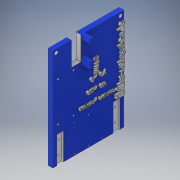
# Autodesk Inventor part: MainBody
Saved by Autodesk Inventor 2018 (Build 220112000, 112)
## iProperties
Created: 2018-10-10
Part Number: MainBody
Material: Generic
Document SubType Name: Modeling
Designer: Viraj Shah
Density: 1 g/cm^3
Appearance: Default
Author: Viraj Shah
Autodesk Inventor part; units mm, degrees
ref_plane "YZ Plane" through (0, 0, 0) normal (1, 0, 0) x (0, 1, 0)
ref_plane "XZ Plane" through (0, 0, 0) normal (0, 1, 0) x (-1, 0, 0)
ref_plane "XY Plane" through (0, 0, 0) normal (0, 0, 1) x (1, 0, 0)
sketch "Sketch1" plane through (0, 0, 0) normal (1, 0, 0) x (0, 1, 0)
  line L0 (50, -400.7355) -> (-50, -400.7355)
  line L1 (-50, -400.7355) -> (-50, -430.7355)
  line L2 (-50, -430.7355) -> (50, -430.7355)
  line L3 (50, -430.7355) -> (50, -400.7355)
  line L4 (-52.5, -305.7355) -> (52.5, -305.7355)
  line L5 (52.5, -305.7355) -> (52.5, -455.7355)
  line L6 (52.5, -455.7355) -> (-52.5, -455.7355)
  line L7 (-52.5, -455.7355) -> (-52.5, -305.7355)
  dimension "d4" = 100
  dimension "d5" = 30
  dimension "d7" = 105
  dimension "d8" = 150
  dimension "d9" = 2.5
  dimension "d10" = 55
  constraints: 16 end point, 4 parallel, 2 perpendicular, 1 horizontal
  measures "d4" distance of L3.start L2.start
  measures "d5" distance of L2.start L0.end
  measures "d7" distance of L5.end L6.end
  measures "d8" distance of L4.end L5.end
  measures "d9" distance between parallel lines of L7 L1
  measures "d10" distance between parallel lines of L6 L0
extrude "Extrusion1" add sketch "Sketch1" along normal blind 7 contours L3 L2 L1 L0 | L4 L5 L6 L7
sketch "Sketch3" plane through (0, -52.5, -455.7355) normal (0, 0, -1) x (-1, 0, 0)
  line L0 (0, 0) -> (-7, 0) projected
  line L1 (-7, 0) -> (-7, 105) projected
  line L2 (-7, 6) -> (-4.5, 6)
  line L3 (-4.5, 6) -> (-4.5, 16)
  line L4 (-4.5, 16) -> (-7, 16)
  line L5 (-7, 6) -> (-7, 16)
  line L6 (0, 52.5) -> (-22.4318, 52.5)
  line L7 (-7, 99) -> (-4.5, 99)
  line L8 (-4.5, 99) -> (-4.5, 89)
  line L9 (-4.5, 89) -> (-7, 89)
  line L10 (-7, 99) -> (-7, 89)
  dimension "d19" = 6
  dimension "d20" = 2.5
  dimension "d21" = 10
  constraints: 18 end point, 4 symmetric about line, 2 horizontal, 2 perpendicular, 2 point on line
  measures "d19" distance of L0.end L2.start
  measures "d20" distance of L2.start L2.end
  measures "d21" distance of L2.end L3.end
extrude "Extrusion3" cut sketch "Sketch3" against normal blind 40
sketch "Sketch4" plane through (7, 0, 0) normal (1, 0, 0) x (0, 0, -1)
  line L0 (305.7355, -52.5) -> (455.7355, -52.5) projected
  line L1 (305.7355, 52.5) -> (305.7355, -52.5) projected
  line L2 (455.7355, 52.5) -> (305.7355, 52.5) projected
  circle A0 centre (310.7355, 47.5) radius 2.5
  circle A1 centre (310.7355, -47.5) radius 2.5
  point P0 (0, 0)
  dimension "d24" = 5
  dimension "d25" = 5
  dimension "d26" = 5
  dimension "d27" = 5
  dimension "d28" = 5
  dimension "d29" = 5
  constraints: 2 centre point, 2 coincident
  measures "d24" distance from line of L0 point (310.736, -47.5)
  measures "d25" distance from line of L1 point (310.736, -47.5)
  measures "d26" distance from line of L2 point (310.736, 47.5)
  measures "d27" distance from line of L1 point (310.736, 47.5)
  measures "d28" diameter of A0
  measures "d29" diameter of A1
extrude "Extrusion4" cut sketch "Sketch4" against normal blind 40
sketch "Sketch5" plane through (7, 0, 0) normal (1, 0, 0) x (0, 0, -1)
  line L0 (305.7355, -52.5) -> (455.7355, -52.5) projected
  line L1 (305.7355, 52.5) -> (305.7355, -52.5) projected
  circle A0 centre (345.7355, -44.85) radius 1.375
  circle A1 centre (345.7355, -21.85) radius 1.375
  circle A2 centre (403.7355, -21.85) radius 1.375
  circle A3 centre (403.7355, -44.85) radius 1.375
  point P0 (0, 0)
  dimension "d32" = 23
  dimension "d34" = 58
  dimension "d35" = 7.65
  dimension "d36" = 7.65
  dimension "d37" = 0
  dimension "d38" = 58
  dimension "d39" = 40
  dimension "d40" = 2.75
  dimension "d41" = 2.75
  dimension "d42" = 2.75
  dimension "d43" = 2.75
  dimension "d111" = 23
  constraints: 4 centre point, 4 coincident
  measures "d32" distance of point (345.736, -21.85) point (345.736, -44.85)
  measures "d34" distance of point (345.736, -44.85) point (403.736, -44.85)
  measures "d35" distance from line of L0 point (345.736, -44.85)
  measures "d36" distance from line of L0 point (403.736, -44.85)
  measures "d37" horizontal distance of point (403.736, -21.85) point (403.736, -44.85)
  measures "d38" distance of point (403.736, -21.85) point (345.736, -21.85)
  measures "d39" distance from line of L1 point (345.736, -21.85)
  measures "d40" diameter of A0
  measures "d41" diameter of A1
  measures "d42" diameter of A2
  measures "d43" diameter of A3
  measures "d111" distance of point (403.736, -21.85) point (403.736, -44.85)
extrude "Extrusion5" cut sketch "Sketch5" against normal blind 40
sketch "Sketch6" plane through (7, 0, 0) normal (1, 0, 0) x (0, 0, -1)
  line L0 (0, 0) -> (765.3396, 0)
  line L1 (305.7355, -25) -> (340.7355, -25)
  line L2 (305.7355, -11) -> (340.7355, -11)
  line L3 (340.7355, -11) -> (340.7355, -25)
  line L4 (305.7355, -25) -> (305.7355, -11)
  constraints: 10 end point, 1 horizontal
extrude "Extrusion6" cut sketch "Sketch6" against normal blind 40
sketch "Sketch7" plane through (7, 0, 0) normal (1, 0, 0) x (0, 0, -1)
  line L0 (305.7355, 52.5) -> (305.7355, -11) projected
  line L1 (305.7355, -10) -> (311.7355, -10)
  line L2 (311.7355, -10) -> (311.7355, -5)
  line L3 (311.7355, -5) -> (305.7355, -5)
  line L4 (305.7355, -5) -> (305.7355, -10)
  line L5 (305.7355, -11) -> (340.7355, -11) projected
  line L6 (335.2355, -10) -> (344.2355, -10)
  line L7 (344.2355, -10) -> (344.2355, -5)
  line L8 (344.2355, -5) -> (335.2355, -5)
  line L9 (335.2355, -5) -> (335.2355, -10)
  point P0 (0, 0)
  dimension "d54" = 6
  dimension "d55" = 5
  dimension "d56" = 1
  dimension "d57" = 9
  dimension "d58" = 5
  dimension "d59" = 23.5
  dimension "d73" = 0
  constraints: 16 end point, 4 parallel, 2 horizontal, 2 perpendicular, 1 point on line
  measures "d54" distance of L3.end L2.end
  measures "d55" distance of L2.end L1.end
  measures "d56" distance between parallel lines of L5 L1
  measures "d57" distance of L8.end L7.end
  measures "d58" distance of L7.end L6.end
  measures "d59" distance between parallel lines of L9 L2
  measures "d73" distance between parallel lines of L6 L1
extrude "Extrusion7" add sketch "Sketch7" along normal blind 12
sketch "Sketch8" plane through (7, -10, -344.2355) normal (0, -1, 0) x (1, 0, 0)
  line L0 (12, 38.5) -> (12, 32.5) projected
  line L1 (12, 9) -> (12, 0) projected
  line L2 (0, 9) -> (12, 9) projected
  point P0 (-7, 344.2355)
  point P1 (6, 6.5)
  point P2 (6, 35.5)
  dimension "d62" = 6
  dimension "d63" = 6
  dimension "d64" = 2.5
  dimension "d65" = 29
  measures "d62" distance from line of L0 point (6, 35.5)
  measures "d63" distance from line of L1 point (6, 6.5)
  measures "d64" distance from line of L2 point (6, 6.5)
  measures "d65" distance of point (6, 35.5) point (6, 6.5)
hole "Hole1" [suppressed]
sketch "Sketch10" plane through (4.5, -46.5, -455.7355) normal (1, 0, 0) x (0, 0, -1)
  line L0 (0, 0) -> (-40, 0) projected
  line L1 (0, 99) -> (0, -6) projected
  circle A0 centre (-30, 5) radius 1
  circle A1 centre (-10, 5) radius 1
  line L2 (0, 10) -> (0, 83) projected
  line L3 (0, 46.5) -> (-66.3883, 46.5)
  circle A2 centre (-30, 88) radius 1
  circle A3 centre (-10, 88) radius 1
  point P0 (-455.7355, 46.5)
  dimension "d77" = 2
  dimension "d78" = 2
  constraints: 4 centre point, 4 coincident, 4 symmetric about line, 2 end point, 1 horizontal, 1 midpoint, 2 other
  measures "d77" diameter of A0
  measures "d78" diameter of A1
extrude "Extrusion8" cut sketch "Sketch10" against normal blind 10
sketch "Sketch11" plane through (7, 0, 0) normal (1, 0, 0) x (0, 0, -1)
  circle A0 centre (369.0216, 10.3693) radius 3.1
  circle A1 centre (384.0216, 10.3693) radius 3.1
  circle A2 centre (399.0216, 10.3693) radius 3.1
  point P0 (0, 0)
  dimension "d83" = 15
  dimension "d84" = 15
  dimension "d85" = 6.2
  dimension "d86" = 6.2
  dimension "d87" = 6.2
  constraints: 3 centre point, 3 coincident
  measures "d83" distance of point (384.022, 10.369) point (369.022, 10.369)
  measures "d84" distance of point (384.022, 10.369) point (399.022, 10.369)
  measures "d85" diameter of A0
  measures "d86" diameter of A1
  measures "d87" diameter of A2
extrude "Extrusion9" cut sketch "Sketch11" against normal blind 10
sketch "Sketch12" plane through (7, 0, 0) normal (1, 0, 0) x (0, 0, -1)
  line L0 (305.7355, 52.5) -> (455.7355, 52.5) projected
  line L1 (389.0354, 35.8376) -> (378.0354, 35.8376)
  line L2 (378.0354, 38.8376) -> (382.0354, 38.8376)
  line L3 (382.0354, 38.8376) -> (382.0354, 47.8376)
  line L4 (382.0354, 47.8376) -> (378.0354, 47.8376)
  line L5 (389.0354, 38.8376) -> (385.0354, 38.8376)
  line L6 (385.0354, 38.8376) -> (385.0354, 47.8376)
  line L7 (385.0354, 47.8376) -> (389.0354, 47.8376)
  line L8 (373.0515, 35.8462) -> (373.0946, 50.8376)
  line L9 (370.0702, 42.3462) -> (364.3334, 35.8376)
  line L10 (364.3334, 35.8376) -> (362.9588, 37.6685)
  line L11 (370.0759, 44.3462) -> (364.3766, 50.8877)
  line L12 (364.3766, 50.8877) -> (362.9915, 49.0648)
  line L13 (370.0515, 35.8462) -> (370.0702, 42.3462)
  line L14 (370.0759, 44.3462) -> (370.0946, 50.8462)
  line L15 (362.3922, 38.3188) -> (366.8317, 43.3555)
  line L16 (366.8317, 43.3555) -> (362.4632, 48.3694)
  line L17 (369.2394, 50.8376) -> (369.2395, 50.8487)
  line L18 (362.9915, 49.0648) -> (362.4632, 48.3694)
  line L19 (362.9588, 37.6685) -> (362.3922, 38.3188)
  line L20 (347.6585, 38.8376) -> (351.6582, 38.8376)
  line L21 (351.6582, 38.8376) -> (351.6582, 47.8376)
  line L22 (351.6582, 47.8376) -> (347.6585, 47.8376)
  line L23 (358.6585, 38.8376) -> (354.6582, 38.8376)
  line L24 (354.6582, 38.8376) -> (354.6582, 47.8376)
  line L25 (354.6582, 47.8376) -> (358.6585, 47.8376)
  line L26 (391.0354, 35.8376) -> (391.0354, 35.8462)
  line L27 (378.0354, 50.8376) -> (389.0354, 50.8376)
  line L28 (370.0945, 50.8376) -> (373.0946, 50.8376)
  line L29 (364.3386, 50.8376) -> (364.4202, 50.8376)
  line L30 (389.0354, 35.8376) -> (378.0354, 35.8376)
  line L31 (373.0515, 35.8462) -> (370.0515, 35.8462)
  line L32 (358.6585, 35.8376) -> (347.6585, 35.8376)
  line L33 (358.6585, 50.8376) -> (347.6585, 50.8376)
  line L34 (389.0354, 35.8376) -> (389.0354, 38.8376)
  line L35 (389.0354, 47.8376) -> (389.0354, 50.8376)
  line L36 (378.0354, 35.8376) -> (378.0354, 38.8376)
  line L37 (378.0354, 47.8376) -> (378.0354, 50.8376)
  line L38 (376.0354, 35.8376) -> (376.0354, 35.8462)
  line L39 (358.6585, 35.8376) -> (358.6585, 38.8376)
  line L40 (358.6585, 47.8376) -> (358.6585, 50.8376)
  line L41 (347.6585, 35.8376) -> (347.6585, 38.8376)
  line L42 (347.6585, 47.8376) -> (347.6585, 50.8376)
  point P0 (0, 0)
  constraints: 84 end point, 14 parallel, 7 perpendicular, 5 point on line, 3 horizontal
extrude "Extrusion10" [suppressed]
sketch "Sketch14" plane through (7, 0, 0) normal (1, 0, 0) x (0, 0, -1)
  circle A0 centre (399.0216, 10.3693) radius 3.1 projected
  line L0 (383.5696, 16.8077) -> (384.0734, 16.8077) construction
  line L1 (383.5696, 14.7372) -> (384.0734, 14.7372)
  line L2 (384.0734, 18.8783) -> (383.5696, 18.8783)
  arc A1 (383.5696, 18.8783) -> (383.5696, 14.7372) centre (383.5696, 16.8077) ccw
  arc A2 (384.0734, 14.7372) -> (384.0734, 18.8783) centre (384.0734, 16.8077) ccw
  line L3 (384.0734, 16.1243) -> (383.5696, 16.1243)
  arc A3 (383.5696, 17.4911) -> (383.5696, 16.1243) centre (383.5696, 16.8077) ccw
  line L4 (383.5696, 17.4911) -> (384.0734, 17.4911)
  arc A4 (384.0734, 16.1243) -> (384.0734, 17.4911) centre (384.0734, 16.8077) ccw
  line L5 (386.247, 19.4647) -> (381.907, 19.4647)
  line L6 (386.247, 20.5147) -> (383.3413, 20.5147)
  line L7 (381.907, 20.7247) -> (384.4441, 22.1895)
  line L8 (386.1241, 22.1895) -> (384.5223, 21.2647)
  line L9 (386.1241, 23.2395) -> (381.802, 23.2395)
  line L10 (384.4441, 22.1895) -> (381.802, 22.1895)
  line L11 (384.5223, 21.2647) -> (383.3413, 20.5147)
  line L12 (386.247, 19.4647) -> (386.247, 20.5147)
  line L13 (386.1241, 22.1895) -> (386.1241, 23.2395)
  line L14 (381.907, 19.4647) -> (381.907, 20.7247)
  line L15 (381.802, 22.1895) -> (381.802, 23.2395)
  circle A5 centre (384.0216, 10.3693) radius 3.1 projected
  line L16 (386.1316, 3.7704) -> (381.4806, 3.7704)
  line L17 (381.4806, 6.4304) -> (382.3206, 6.4304)
  line L18 (382.3206, 6.4304) -> (382.3206, 4.6104)
  line L19 (382.3206, 4.6104) -> (383.1606, 4.6104)
  line L20 (383.1606, 4.6104) -> (383.1606, 5.8704)
  line L21 (384.0006, 5.8704) -> (384.0006, 4.6104)
  line L22 (384.0006, 4.6104) -> (386.1316, 4.6104)
  line L23 (386.1316, 3.7704) -> (386.1316, 4.6104)
  line L24 (381.4806, 6.4304) -> (381.4806, 3.7704)
  line L25 (383.1606, 5.8704) -> (384.0006, 5.8704)
  line L26 (381.4806, 3.4273) -> (382.3206, 3.4273)
  line L27 (382.3206, 1.6073) -> (383.1606, 1.6073)
  line L28 (384.0006, 2.8673) -> (384.0006, 1.6073)
  line L29 (383.1606, 1.6073) -> (383.1606, 2.8673)
  line L30 (382.3206, 3.4273) -> (382.3206, 1.6073)
  line L31 (384.0006, 1.6073) -> (386.1316, 1.6073)
  line L32 (386.1316, 0.7673) -> (381.4806, 0.7673)
  line L33 (386.1316, 0.7673) -> (386.1316, 1.6073)
  line L34 (381.4806, 3.4273) -> (381.4806, 0.7673)
  line L35 (383.1606, 2.8673) -> (384.0006, 2.8673)
  line L36 (397.327, -12.2248) -> (397.975, -12.2248)
  line L37 (397.975, -13.6288) -> (398.623, -13.6288)
  line L38 (399.271, -12.6568) -> (399.271, -13.6288)
  line L39 (398.623, -13.6288) -> (398.623, -12.6568)
  line L40 (397.975, -12.2248) -> (397.975, -13.6288)
  line L41 (399.271, -13.6288) -> (400.9149, -13.6288)
  line L42 (400.9149, -14.2768) -> (397.327, -14.2768)
  line L43 (400.9149, -14.2768) -> (400.9149, -13.6288)
  line L44 (397.327, -12.2248) -> (397.327, -14.2768)
  line L45 (398.623, -12.6568) -> (399.271, -12.6568)
  line L46 (400.9651, -8.0846) -> (397.2712, -8.0846)
  arc A6 (399.1232, -6.8327) -> (397.2712, -6.8342) centre (398.1975, -7.1989) ccw
  line L47 (399.1232, -6.8327) -> (401.0087, -6.0517)
  line L48 (399.374, -7.3782) -> (401.0087, -6.7011)
  line L49 (400.9651, -7.4846) -> (399.374, -7.4846)
  line L50 (399.374, -7.3782) -> (399.374, -7.4846)
  line L51 (397.297, -5.8571) -> (400.9651, -5.8571)
  line L52 (397.297, -5.2571) -> (400.4972, -5.2571)
  line L53 (400.9651, -4.8344) -> (399.5174, -3.9985)
  line L54 (400.9651, -4.8344) -> (402.6367, -4.8344) construction
  line L55 (400.4972, -5.2571) -> (398.2454, -3.957)
  line L56 (397.297, -2.1024) -> (400.9651, -2.1024)
  line L57 (397.297, -2.6569) -> (400.4972, -2.6569)
  line L58 (400.9651, -3.1627) -> (399.5174, -3.9985)
  line L59 (400.4972, -2.6569) -> (398.2454, -3.957)
  line L60 (400.9651, -1.8466) -> (397.327, -0.3767)
  line L61 (400.9651, -1.2642) -> (399.6523, -0.7338)
  line L62 (400.9651, 0.8232) -> (397.327, -0.3767)
  line L63 (400.9651, 0.2546) -> (399.6523, -0.1784)
  line L64 (399.6523, -0.7338) -> (399.6523, -0.1784)
  line L65 (400.9371, 1.2698) -> (397.2991, 1.2698)
  arc A7 (399.1511, 2.5217) -> (397.2991, 2.5201) centre (398.2254, 2.1554) ccw
  line L66 (399.1511, 2.5217) -> (401.0366, 3.3027)
  line L67 (399.4019, 1.9761) -> (401.0366, 2.6532)
  line L68 (400.9371, 1.8698) -> (399.4019, 1.8698)
  line L69 (399.4019, 1.9761) -> (399.4019, 1.8698)
  line L70 (400.9651, 3.7854) -> (397.327, 3.7854)
  arc A8 (400.9651, 3.7854) -> (397.327, 3.7854) centre (399.146, 4.0442) ccw
  line L71 (400.9651, -8.0846) -> (400.9651, -7.4846)
  line L72 (401.0087, -6.7011) -> (401.0087, -6.0517)
  line L73 (400.9651, -5.8571) -> (400.9651, -4.8344)
  line L74 (400.9651, -3.1627) -> (400.9651, -2.1024)
  line L75 (400.9651, -1.8466) -> (400.9651, -1.2642)
  line L76 (400.9651, 0.2546) -> (400.9651, 0.8232)
  line L77 (400.9371, 1.2698) -> (400.9371, 1.8698)
  line L78 (401.0366, 2.6532) -> (401.0366, 3.3027)
  line L79 (397.2712, -8.0846) -> (397.2712, -6.8342)
  line L80 (397.297, -5.8571) -> (397.297, -5.2571)
  line L81 (397.297, -2.6569) -> (397.297, -2.1024)
  line L82 (397.2991, 1.2698) -> (397.2991, 2.5201)
  line L83 (397.3471, 24.6024) -> (401.0152, 24.6024)
  line L84 (397.3471, 25.2024) -> (400.5474, 25.2024)
  line L85 (401.0152, 25.6252) -> (399.5675, 26.461)
  line L86 (401.0152, 25.6252) -> (402.6869, 25.6252) construction
  line L87 (400.5474, 25.2024) -> (398.2955, 26.5026)
  line L88 (397.3471, 28.3572) -> (401.0152, 28.3572)
  line L89 (397.3471, 27.8027) -> (400.5474, 27.8027)
  line L90 (400.5474, 27.8027) -> (398.2955, 26.5026)
  line L91 (401.0152, 27.2968) -> (399.5675, 26.461)
  line L92 (401.0152, 28.613) -> (397.3771, 30.0828)
  line L93 (401.0152, 29.1954) -> (399.7025, 29.7257)
  line L94 (401.0152, 31.2828) -> (397.3771, 30.0828)
  line L95 (401.0152, 30.7142) -> (399.7025, 30.2812)
  line L96 (399.7025, 29.7257) -> (399.7025, 30.2812)
  arc A9 (399.2012, 32.7656) -> (397.3492, 32.764) centre (398.2755, 32.3993) ccw
  line L97 (399.4521, 32.22) -> (399.4521, 32.1137)
  line L98 (400.9873, 31.5137) -> (397.3492, 31.5137)
  line L99 (399.2012, 32.7656) -> (401.0867, 33.5466)
  line L100 (399.4521, 32.22) -> (401.0867, 32.8971)
  line L101 (400.9873, 32.1137) -> (399.4521, 32.1137)
  line L102 (401.0152, 34.2449) -> (397.3771, 34.2449)
  arc A10 (401.0152, 34.2449) -> (397.3771, 34.2449) centre (399.1962, 34.5038) ccw
  line L103 (401.0152, 24.6024) -> (401.0152, 25.6252)
  line L104 (401.0152, 27.2968) -> (401.0152, 28.3572)
  line L105 (401.0152, 28.613) -> (401.0152, 29.1954)
  line L106 (401.0152, 30.7142) -> (401.0152, 31.2828)
  line L107 (400.9873, 31.5137) -> (400.9873, 32.1137)
  line L108 (401.0867, 32.8971) -> (401.0867, 33.5466)
  line L109 (397.3471, 24.6024) -> (397.3471, 25.2024)
  line L110 (397.3471, 27.8027) -> (397.3471, 28.3572)
  line L111 (397.3492, 31.5137) -> (397.3492, 32.764)
  arc A11 (399.1962, 16.0661) -> (397.3771, 16.0699) centre (398.286, 15.7439) ccw
  line L112 (397.3771, 14.8176) -> (397.3771, 16.0699)
  line L113 (399.1962, 14.8176) -> (397.3771, 14.8176)
  line L114 (399.1962, 14.8176) -> (401.0152, 14.8176)
  arc A12 (401.0152, 16.0699) -> (399.1962, 16.0661) centre (400.1064, 15.7439) ccw
  line L115 (401.0152, 16.7094) -> (401.0152, 17.2918)
  line L116 (401.0152, 16.7094) -> (397.3771, 18.1793)
  line L117 (401.0152, 17.2918) -> (399.7025, 17.8222)
  line L118 (401.0152, 19.3792) -> (397.3771, 18.1793)
  line L119 (401.0152, 18.8106) -> (399.7025, 18.3776)
  line L120 (399.7025, 17.8222) -> (399.7025, 18.3776)
  line L121 (401.0152, 18.8106) -> (401.0152, 19.3792)
  arc A13 (397.4543, 21.4637) -> (400.9493, 21.4059) centre (399.1937, 20.9472) ccw
  arc A14 (398.3792, 20.9472) -> (400.0082, 20.9472) centre (399.1937, 20.9472) ccw
  line L122 (398.3792, 20.9472) -> (398.3792, 21.4637)
  line L123 (400.0082, 20.9472) -> (400.0082, 21.4059)
  line L124 (397.4543, 21.4637) -> (398.3792, 21.4637)
  line L125 (400.0082, 21.4059) -> (400.9493, 21.4059)
  line L126 (397.3771, 21.9899) -> (401.0152, 21.9899)
  line L127 (398.6702, 22.5899) -> (397.3771, 23.883)
  line L128 (397.8014, 24.3073) -> (399.3091, 22.7996)
  line L129 (399.948, 22.5899) -> (401.0152, 23.6571)
  line L130 (400.5909, 24.0814) -> (399.3091, 22.7996)
  line L131 (397.3771, 22.5899) -> (398.6702, 22.5899)
  line L132 (399.948, 22.5899) -> (401.0152, 22.5899)
  line L133 (401.0152, 23.6571) -> (400.5909, 24.0814)
  line L134 (397.3771, 23.883) -> (397.8014, 24.3073)
  line L135 (401.0152, 22.5899) -> (401.0152, 21.9899)
  line L136 (397.3771, 22.5899) -> (397.3771, 21.9899)
  circle A15 centre (369.0216, 10.3693) radius 3.1 projected
  line L137 (365.9216, 23.083) -> (365.9216, 23.9821)
  line L138 (368.4931, 16.6306) -> (369.1625, 16.6306) construction
  line L139 (368.5036, 14.5059) -> (369.173, 14.5092)
  line L140 (369.152, 18.7587) -> (368.4826, 18.7554)
  line L141 (368.4897, 17.3185) -> (369.03, 17.3212)
  line L142 (369.0055, 15.9453) -> (368.4965, 15.9428)
  arc A16 (368.4897, 17.3185) -> (368.4965, 15.9428) centre (368.4931, 16.6306) ccw
  arc A17 (369.0055, 15.9453) -> (369.03, 17.3212) centre (369.1625, 16.6306) ccw
  arc A18 (368.4826, 18.7554) -> (368.5036, 14.5059) centre (368.4931, 16.6306) ccw
  arc A19 (369.173, 14.5092) -> (371.2812, 16.5222) centre (369.1625, 16.6306) ccw
  arc A20 (370.9611, 17.7681) -> (369.152, 18.7587) centre (369.1625, 16.6306) ccw
  line L143 (371.2812, 16.5222) -> (372.4335, 18.518)
  line L144 (371.2812, 16.5222) -> (373.5859, 16.5222) construction
  line L145 (370.9611, 17.7681) -> (371.8272, 19.2681)
  line L146 (370.9611, 17.7681) -> (372.6932, 17.7681) construction
  line L147 (372.4335, 18.518) -> (371.8272, 19.2681)
  line L148 (372.1216, 19.9028) -> (365.9216, 23.083)
  line L149 (372.1216, 23.9686) -> (369.7794, 22.0033)
  line L150 (372.1216, 24.3698) -> (374.6501, 24.3698) construction
  line L151 (372.1216, 25.0129) -> (369.007, 22.3995)
  line L152 (372.1216, 19.9028) -> (372.1216, 20.8019)
  line L153 (372.1216, 23.9686) -> (372.1216, 25.0129)
  line L154 (372.1216, 20.8019) -> (369.7794, 22.0033)
  line L155 (369.007, 22.3995) -> (365.9216, 23.9821)
  arc A21 (368.8932, 3.7279) -> (368.9, 2.3522) centre (368.8966, 3.0401) ccw
  line L156 (368.9071, 0.9153) -> (369.5765, 0.9186)
  line L157 (369.409, 2.3547) -> (368.9, 2.3522)
  line L158 (368.8966, 3.0401) -> (369.566, 3.0401) construction
  line L159 (368.8932, 3.7279) -> (369.4335, 3.7306)
  arc A22 (369.409, 2.3547) -> (369.4335, 3.7306) centre (369.566, 3.0401) ccw
  arc A23 (368.8861, 5.1648) -> (368.9071, 0.9153) centre (368.8966, 3.0401) ccw
  line L160 (369.5555, 5.1681) -> (368.8861, 5.1648)
  line L161 (372.5251, 4.42) -> (372.5251, 5.4504)
  arc A24 (369.5765, 0.9186) -> (371.6847, 2.9316) centre (369.566, 3.0401) ccw
  arc A25 (371.3646, 4.1775) -> (369.5555, 5.1681) centre (369.566, 3.0401) ccw
  line L162 (371.6847, 2.9316) -> (372.837, 4.9274)
  line L163 (371.6847, 2.9316) -> (373.9893, 2.9316) construction
  line L164 (371.3646, 4.1775) -> (372.2306, 5.6775)
  line L165 (371.3646, 4.1775) -> (373.0967, 4.1775) construction
  line L166 (372.837, 4.9274) -> (372.2306, 5.6775)
  line L167 (360.9007, 12.9625) -> (358.6077, 7.2872)
  line L168 (359.9921, 12.9625) -> (359.1647, 10.9147)
  line L169 (356.7358, 12.9625) -> (358.6077, 7.2872)
  line L170 (357.6228, 12.9625) -> (358.2982, 10.9147)
  line L171 (359.1647, 10.9147) -> (358.2982, 10.9147)
  line L172 (360.9007, 12.9625) -> (359.9921, 12.9625)
  line L173 (357.6228, 12.9625) -> (356.7358, 12.9625)
  line L174 (364.5611, 7.2699) -> (363.5675, 12.9956)
  line L175 (363.2589, 7.2699) -> (362.5002, 11.6419)
  line L176 (362.5002, 13.2978) -> (367.8961, 13.2978) construction
  line L177 (360.4301, 7.2764) -> (361.3567, 12.9956)
  line L178 (361.7296, 7.2764) -> (362.5002, 11.6419)
  line L179 (356.3334, 7.2699) -> (356.3334, 12.9956)
  line L180 (352.6489, 12.9956) -> (352.6489, 11.9386)
  line L181 (352.6489, 11.9386) -> (355.12, 11.9386)
  line L182 (355.12, 11.9386) -> (355.12, 7.2699)
  line L183 (355.12, 11.9386) -> (361.2012, 11.9386) construction
  line L184 (351.4679, 7.2699) -> (351.4679, 11.6838)
  line L185 (348.4679, 7.2699) -> (348.4679, 11.6838)
  arc A26 (351.4679, 11.6838) -> (348.4679, 11.6838) centre (349.9679, 11.0315) ccw
  line L186 (347.4679, 7.2699) -> (347.4679, 11.8664)
  arc A27 (352.4679, 11.8664) -> (347.4679, 11.8664) centre (349.9679, 11.0315) ccw
  line L187 (352.4679, 11.8664) -> (352.4679, 7.2699)
  line L188 (343.5709, 7.2699) -> (343.5709, 8.3067)
  line L189 (344.2621, 9.3435) -> (344.2621, 9.9435)
  line L190 (345.8173, 8.3067) -> (345.8173, 9.3435)
  line L191 (345.8173, 9.3435) -> (344.2621, 9.3435)
  line L192 (343.5709, 8.3067) -> (345.8173, 8.3067)
  line L193 (343.5709, 7.2699) -> (346.8539, 7.2699)
  line L194 (346.8539, 10.2699) -> (346.8539, 7.2699)
  line L195 (343.5709, 13.0199) -> (343.5709, 11.9831)
  line L196 (344.2621, 10.5435) -> (344.2621, 9.9435)
  line L197 (345.8173, 11.9831) -> (345.8173, 10.5435)
  line L198 (345.8173, 10.5435) -> (344.2621, 10.5435)
  line L199 (343.5709, 11.9831) -> (345.8173, 11.9831)
  line L200 (343.5709, 13.0199) -> (346.8539, 13.0199)
  line L201 (346.8539, 10.2699) -> (346.8539, 13.0199)
  line L202 (356.3334, 7.2699) -> (355.12, 7.2699)
  line L203 (356.3334, 12.9956) -> (352.6489, 12.9956)
  line L204 (352.4679, 7.2699) -> (351.4679, 7.2699)
  line L205 (348.4679, 7.2699) -> (347.4679, 7.2699)
  line L206 (383.5696, -2.0145) -> (384.0734, -2.0145) construction
  line L207 (383.5696, -4.0851) -> (384.0734, -4.0851)
  line L208 (384.0734, 0.0561) -> (383.5696, 0.0561)
  line L209 (383.5696, -1.3311) -> (384.0734, -1.3311)
  line L210 (384.0734, -2.6979) -> (383.5696, -2.6979)
  arc A28 (383.5696, -1.3311) -> (383.5696, -2.6979) centre (383.5696, -2.0145) ccw
  arc A29 (384.0734, -2.6979) -> (384.0734, -1.3311) centre (384.0734, -2.0145) ccw
  arc A30 (384.0734, -4.0851) -> (384.0734, 0.0561) centre (384.0734, -2.0145) ccw
  arc A31 (383.5696, 0.0561) -> (383.5696, -4.0851) centre (383.5696, -2.0145) ccw
  line L211 (398.8521, -10.4106) -> (399.2803, -10.4106) construction
  line L212 (398.8521, -12.1706) -> (399.2803, -12.1706)
  line L213 (399.2803, -8.6506) -> (398.8521, -8.6506)
  line L214 (398.8521, -9.8297) -> (399.2803, -9.8297)
  line L215 (399.2803, -10.9915) -> (398.8521, -10.9915)
  arc A32 (398.8521, -9.8297) -> (398.8521, -10.9915) centre (398.8521, -10.4106) ccw
  arc A33 (399.2803, -10.9915) -> (399.2803, -9.8297) centre (399.2803, -10.4106) ccw
  arc A34 (399.2803, -12.1706) -> (399.2803, -8.6506) centre (399.2803, -10.4106) ccw
  arc A35 (398.8521, -8.6506) -> (398.8521, -12.1706) centre (398.8521, -10.4106) ccw
  line L216 (401.0152, 14.8176) -> (401.0152, 16.0699)
  line L217 (364.5611, 7.2699) -> (363.2589, 7.2699)
  line L218 (361.7296, 7.2764) -> (360.4301, 7.2764)
  line L219 (363.5675, 12.9956) -> (361.3567, 12.9956)
  point P0 (0, 0)
  point P1 (383.8215, 16.8077)
  point P2 (399.2174, -4.5182)
  point P3 (399.2174, -3.3958)
  point P4 (399.2675, 25.9414)
  point P5 (399.2675, 27.0638)
  point P6 (368.8278, 16.6306)
  point P7 (369.2313, 3.0401)
  point P8 (383.8215, -2.0145)
  point P9 (399.0662, -10.4106)
  dimension "d118" = 1.05
  dimension "d119" = 0.84
  dimension "d120" = 1.05
  dimension "d121" = 30
  dimension "d122" = 30
  dimension "d123" = 1.05
  dimension "d124" = 1.26
  dimension "d132" = 2.66
  dimension "d133" = 0.84
  dimension "d134" = 1.26
  dimension "d135" = 2.66
  dimension "d136" = 0.84
  dimension "d137" = 1.26
  dimension "d138" = 2.052
  dimension "d139" = 0.648
  dimension "d140" = 0.972
  dimension "d147" = 0.6
  dimension "d148" = 0.6
  dimension "d149" = 0.6
  dimension "d151" = 150
  dimension "d152" = 0.6
  dimension "d159" = 0.6
  dimension "d160" = 0.6
  dimension "d168" = 0.6
  dimension "d169" = 150
  dimension "d170" = 0.6
  dimension "d173" = 0.6
  dimension "d174" = 0.6
  dimension "d179" = 1
  dimension "d182" = 0.6
  dimension "d183" = 60
  dimension "d184" = 60
  dimension "d185" = 1.5
  dimension "d188" = 140
  dimension "d189" = 0.8
  dimension "d190" = 60
  dimension "d191" = 60
  dimension "d192" = 1.5
  dimension "d193" = 1.283
  dimension "d195" = 90
  dimension "d197" = 3
  dimension "d198" = 3.283
  dimension "d200" = 1.5552
  dimension "d201" = 0.6
  dimension "d202" = 0.6
  dimension "d203" = 3
  dimension "d204" = 2.75
  dimension "d206" = 1
  dimension "d209" = 0.566
  dimension "d212" = 1.389
  constraints: 450 end point, 66 point on circle, 36 parallel, 36 vertical, 33 centre point, 26 horizontal, 25 tangent, 24 perpendicular, 11 point on line, 6 equal length, 5 midpoint, 2 collinear, 15 other
  measures "d118" distance between parallel lines of L6 L5
  measures "d119" distance between parallel lines of L7 L8
  measures "d120" distance between parallel lines of L9 L10
  measures "d121" angle of L8 L6
  measures "d122" angle of L10 L7
  measures "d123" distance of L8.start L9.start
  measures "d124" distance of L5.end L14.end
  measures "d132" distance of L17.start L16.end
  measures "d133" distance of L16.start L22.end
  measures "d134" distance between parallel lines of L19 L25
  measures "d135" distance of L26.start L32.end
  measures "d136" distance of L33.start L31.end
  measures "d137" distance between parallel lines of L27 L35
  measures "d138" distance of L36.start L44.end
  measures "d139" distance of L43.start L41.end
  measures "d140" distance between parallel lines of L37 L45
  measures "d147" distance between parallel lines of L47 L48
  measures "d148" distance between parallel lines of L49 L46
  measures "d149" distance between parallel lines of L51 L52
  measures "d151" angle of L54 L53
  measures "d152" distance between parallel lines of L53 L55
  measures "d159" distance between parallel lines of L66 L67
  measures "d160" distance between parallel lines of L68 L65
  measures "d168" distance between parallel lines of L83 L84
  measures "d169" angle of L86 L85
  measures "d170" distance between parallel lines of L85 L87
  measures "d173" distance between parallel lines of L99 L100
  measures "d174" distance between parallel lines of L101 L98
  measures "d179" radial gap between concentric circles of A13 A14
  measures "d182" distance between parallel lines of L127 L128
  measures "d183" angle of L144 L143
  measures "d184" angle of L146 L145
  measures "d185" vertical distance of L145.start L145.end
  measures "d188" angle of L149 L150
  measures "d189" distance between parallel lines of L149 L151
  measures "d190" angle of L163 L162
  measures "d191" angle of L165 L164
  measures "d192" vertical distance of L164.start L166.end
  measures "d193" distance between parallel lines of L174 L175
  measures "d195" angle of L182 L183
  measures "d197" distance between parallel lines of L184 L185
  measures "d198" distance of L188.start L193.end
  measures "d200" distance between parallel lines of L190 L189
  measures "d201" distance of L196.start L189.end
  measures "d202" distance of L189.start L189.end
  measures "d203" distance of L194.start L193.end
  measures "d204" distance of L194.start L200.end
  measures "d206" distance between parallel lines of L184 L187
  measures "d209" distance between parallel lines of L46 L213
extrude "Extrusion11" add sketch "Sketch14" along normal blind 3 contours A1 L2 A2 L1 | L5 L14 L7 L10 L15 L9 L13 L8 L11 L6 L12 | L16 L24 L17 L18 L19 L20 L25 L21 L22 L23 | L26 L30 L27 L29 L35 L28 L31 L33 L32 L34 | L36 L40 L37 L39 L45 L38 L41 L43 L42 L44 | L46 L79 A6 L47 L72 L48 L50 L49 L71 | L80 L52 L55 L59 L57 L81 L56 L74 L58 L53 L73 L51 | L60 L62 L76 L63 L64 L61 L75 | L65 L82 A7 L66 L78 L67 L69 L68 L77 | L70 A8 | L109 L84 L87 L90 L89 L110 L88 L104 L91 L85 L103 L83 | L92 L94 L106 L95 L96 L93 L105 | L99 L108 L100 L97 L101 L107 L98 L111 A9 | L102 A10 | A12 L216 L114 L113 L112 A11 | L116 L118 L121 L119 L120 L117 L115 | L124 L122 A14 L123 L125 A13 | L136 L131 L127 L134 L128 L130 L133 L129 L132 L135 L126 | L137 L155 L151 L153 L149 L154 L152 L148 | A18 L140 A20 L145 L147 L143 A19 L139 | A23 L160 A25 L164 L166 L162 A24 L156 | L167 L169 L173 L170 L171 L168 L172 | L217 L175 L178 L218 L177 L219 L174 | L202 L182 L181 L180 L203 L179 | L184 A26 L185 L205 L186 A27 L187 L204 | L188 L192 L190 L191 L189 L196 L198 L197 L199 L195 L200 L201 L194 L193 | A31 L208 A30 L207 | A35 L213 A34 L212
sketch "Sketch13" plane through (7, 0, 0) normal (1, 0, 0) x (0, 0, -1)
  line L0 (412.2613, 50.883) -> (412.2613, 41.883)
  line L1 (412.2613, 41.883) -> (409.5613, 41.883)
  line L2 (409.5613, 41.883) -> (409.5613, 50.883)
  circle A0 centre (410.9113, 39.7323) radius 1.5
  line L3 (408.2113, 50.8778) -> (408.2113, 38.2778)
  line L4 (408.2113, 38.2778) -> (406.4113, 38.2778)
  line L5 (406.4113, 45.967) -> (403.6871, 42.5023)
  line L6 (403.6871, 42.5023) -> (402.4152, 43.5024)
  line L7 (402.4152, 43.5024) -> (404.9584, 46.737)
  line L8 (406.4113, 47.507) -> (403.6871, 50.9716)
  line L9 (403.6871, 50.9716) -> (402.4152, 49.9716)
  line L10 (402.4152, 49.9716) -> (404.9584, 46.737)
  line L11 (401.5152, 50.8778) -> (401.5152, 41.8778)
  line L12 (401.5152, 41.8778) -> (398.8152, 41.8778)
  line L13 (398.8152, 41.8778) -> (398.8152, 50.8778)
  circle A1 centre (400.1652, 39.7323) radius 1.5
  line L14 (406.4113, 38.2778) -> (406.4113, 45.967)
  line L15 (406.4113, 47.507) -> (406.4113, 50.8778)
  circle A2 centre (396.8692, 50.1657) radius 0.7
  line L16 (395.715, 41.0746) -> (394.315, 41.0746)
  arc A3 (391.546, 45.7361) -> (394.315, 46.0983) centre (392.6102, 48.3662) ccw
  line L17 (390.6711, 47.0339) -> (390.6711, 50.8746)
  line L18 (391.7211, 50.8746) -> (391.7211, 48.2957)
  arc A4 (392.7904, 46.9353) -> (394.315, 47.4983) centre (393.1343, 48.3499) ccw
  arc A5 (391.7211, 48.2957) -> (392.7904, 46.9353) centre (393.1211, 48.2957) ccw
  arc A6 (390.6711, 47.0339) -> (391.546, 45.7361) centre (392.0711, 47.0339) ccw
  arc A7 (386.0021, 45.6807) -> (389.9276, 46.2949) centre (387.8854, 46.4954) ccw
  arc A8 (389.4748, 49.3464) -> (387.3821, 49.5297) centre (388.3607, 48.6642) ccw
  arc A9 (387.7664, 48.1134) -> (388.9158, 47.706) centre (389.3662, 50.8023) ccw
  arc A10 (387.3821, 49.5297) -> (387.3197, 49.3833) centre (388.9696, 48.7667) ccw
  arc A11 (389.9276, 46.2949) -> (388.9158, 47.706) centre (388.7422, 46.5132) ccw
  arc A12 (387.3197, 49.3833) -> (387.7664, 48.1134) centre (388.3033, 49.0157) ccw
  arc A13 (387.0482, 46.3373) -> (388.7371, 46.5194) centre (387.8854, 46.4954) ccw
  arc A14 (387.1528, 47.0821) -> (388.7371, 46.5194) centre (389.3662, 50.8023) ccw
  arc A15 (386.1957, 49.8035) -> (387.1528, 47.0821) centre (388.3033, 49.0157) ccw
  arc A16 (386.3508, 50.1493) -> (386.1957, 49.8035) centre (388.9696, 48.7667) ccw
  arc A17 (390.2899, 50.2527) -> (386.3508, 50.1493) centre (388.3607, 48.6642) ccw
  line L19 (390.2899, 50.2527) -> (389.4748, 49.3464)
  line L20 (387.0482, 46.3373) -> (386.0021, 45.6807)
  line L21 (385.4307, 47.7809) -> (382.6307, 47.7809)
  line L22 (382.6307, 47.7809) -> (382.6307, 48.8309)
  line L23 (382.6307, 48.8309) -> (385.4307, 48.8309)
  line L24 (385.4307, 48.8309) -> (385.4307, 47.7809)
  line L25 (381.0197, 44.6682) -> (381.0894, 50.8671)
  line L26 (380.0197, 44.6682) -> (380.0718, 49.3006)
  line L27 (379.9448, 50.8671) -> (382.7608, 50.8671) construction
  line L28 (375.0704, 44.7218) -> (375.1276, 50.8995)
  line L29 (376.0704, 44.7218) -> (376.1133, 49.3498)
  line L30 (381.0197, 44.6682) -> (380.0197, 44.6682)
  line L31 (376.0704, 44.7218) -> (375.0704, 44.7218)
  arc A18 (371.5731, 43.9722) -> (374.4386, 46.4824) centre (371.3856, 47.0769) ccw
  arc A19 (374.4386, 46.4824) -> (371.0224, 50.8652) centre (370.8224, 47.1866) ccw
  arc A20 (371.0224, 50.8652) -> (368.3855, 49.9494) centre (370.8225, 47.1867) ccw
  arc A21 (368.9945, 47.0328) -> (371.5731, 43.9722) centre (371.4227, 46.4621) ccw
  arc A22 (370.9726, 49.9497) -> (368.9366, 49.2116) centre (370.8225, 47.1867) ccw
  line L32 (370.2698, 48.0431) -> (373.4538, 48.0431)
  arc A23 (370.2698, 48.0431) -> (368.9945, 47.0328) centre (370.2698, 46.7331) ccw
  arc A24 (373.4538, 48.0431) -> (370.9726, 49.9497) centre (370.8224, 47.1866) ccw
  line L33 (368.9366, 49.2116) -> (368.3855, 49.9494)
  line L34 (366.2691, 43.8649) -> (366.2691, 50.8649)
  line L35 (368.0691, 50.8649) -> (368.0691, 43.8649)
  line L36 (368.0691, 43.8649) -> (366.2691, 43.8649)
  circle A25 centre (367.1274, 42.5122) radius 0.9
  line L37 (364.8448, 50.8649) -> (364.8448, 45.4255)
  arc A26 (360.6758, 45.7361) -> (363.4448, 46.0983) centre (361.74, 48.3662) ccw
  line L38 (359.8009, 47.0339) -> (359.8009, 50.8649)
  line L39 (360.8509, 50.8649) -> (360.8509, 48.2957)
  arc A27 (361.9202, 46.9353) -> (363.4448, 47.4983) centre (362.2641, 48.3499) ccw
  line L40 (363.4448, 45.4255) -> (363.4448, 46.0983)
  line L41 (363.4448, 47.4983) -> (363.4448, 50.8649)
  arc A28 (360.8509, 48.2957) -> (361.9202, 46.9353) centre (362.2509, 48.2957) ccw
  arc A29 (359.8009, 47.0339) -> (360.6758, 45.7361) centre (361.2009, 47.0339) ccw
  line L42 (364.8448, 45.4255) -> (363.4448, 45.4255)
  arc A30 (357.7616, 45.5133) -> (357.9152, 49.0856) centre (356.7226, 47.3474) ccw
  arc A31 (356.1799, 45.4367) -> (357.7616, 45.5133) centre (356.8934, 47.0715) ccw
  arc A32 (355.0907, 46.8116) -> (356.1799, 45.4367) centre (356.8296, 47.0703) ccw
  line L43 (355.0907, 46.8116) -> (355.0907, 50.9583)
  arc A33 (356.1579, 52.1839) -> (355.0907, 50.9583) centre (356.7848, 50.5606) ccw
  arc A34 (359.3268, 50.0608) -> (356.1579, 52.1839) centre (357.1904, 50.2986) ccw
  arc A35 (357.3505, 46.4104) -> (356.9785, 48.446) centre (356.7226, 47.3474) ccw
  arc A36 (356.5571, 46.3415) -> (357.3505, 46.4104) centre (356.8934, 47.0715) ccw
  arc A37 (356.0704, 46.9002) -> (356.5571, 46.3415) centre (356.8296, 47.0703) ccw
  arc A38 (356.9785, 48.446) -> (356.0813, 48.446) centre (356.5299, 43.1844) ccw
  arc A39 (357.9152, 49.0856) -> (356.0647, 49.3355) centre (356.4109, 44.9234) ccw
  line L44 (356.0704, 46.9002) -> (356.0813, 48.446)
  line L45 (356.0647, 49.3355) -> (356.0889, 50.8746)
  arc A40 (352.6906, 48.41) -> (352.9799, 49.9978) centre (352.491, 49.2666) ccw
  arc A41 (352.3665, 50.0499) -> (351.8302, 49.5583) centre (352.4512, 49.4192) ccw
  line L46 (351.8302, 49.5583) -> (351.8302, 48.3487)
  arc A42 (351.8302, 48.3487) -> (352.6906, 48.41) centre (351.9695, 52.4653) ccw
  arc A43 (353.4211, 47.9111) -> (353.3005, 50.6975) centre (352.491, 49.2666) ccw
  arc A44 (353.3005, 50.6975) -> (351.9371, 50.6882) centre (352.6271, 49.4806) ccw
  arc A45 (351.9371, 50.6882) -> (351.861, 50.6547) centre (352.4512, 49.4192) ccw
  arc A46 (352.9799, 49.9978) -> (352.3665, 50.0499) centre (352.6271, 49.4806) ccw
  arc A47 (351.9908, 47.7238) -> (353.4211, 47.9111) centre (352.2678, 51.1647) ccw
  line L47 (351.9908, 47.7238) -> (351.9908, 46.4438)
  arc A48 (351.9908, 46.4438) -> (352.0046, 46.4316) centre (352.2773, 46.756) ccw
  arc A49 (352.0046, 46.4316) -> (353.0962, 46.4379) centre (352.5466, 47.0879) ccw
  arc A50 (351.0966, 46.1356) -> (352.0752, 45.4377) centre (352.2773, 46.756) ccw
  arc A51 (356.2068, 51.0594) -> (356.0889, 50.8746) centre (356.7848, 50.5606) ccw
  arc A52 (358.411, 50.0608) -> (356.2068, 51.0594) centre (357.1904, 50.2986) ccw
  line L48 (359.3268, 50.0608) -> (358.411, 50.0608)
  line L49 (353.0962, 46.4379) -> (353.9199, 47.0246)
  line L50 (353.6516, 45.8487) -> (354.3607, 46.4057)
  arc A53 (352.0752, 45.4377) -> (353.6516, 45.8487) centre (352.3652, 47.5539) ccw
  line L51 (351.861, 50.6547) -> (351.861, 50.8032)
  line L52 (351.861, 50.8032) -> (351.0966, 50.8032)
  line L53 (353.9199, 47.0246) -> (354.3607, 46.4057)
  line L54 (350.4704, 50.8746) -> (350.4704, 45.2746)
  line L55 (350.4704, 45.2746) -> (349.0704, 45.2746)
  arc A54 (347.6132, 45.699) -> (349.0704, 45.7617) centre (348.2723, 47.3456) ccw
  arc A55 (347.6132, 46.2929) -> (349.0704, 46.4438) centre (348.2576, 47.1819) ccw
  line L56 (347.6132, 46.2929) -> (347.6132, 45.699)
  line L57 (349.0704, 45.2746) -> (349.0704, 45.4377)
  line L58 (349.0704, 46.4438) -> (349.0704, 50.8746)
  line L59 (349.0704, 45.7617) -> (349.0704, 45.4255)
  line L60 (346.8371, 41.5185) -> (345.6371, 41.5185)
  line L61 (345.6371, 47.3004) -> (344.7305, 47.3004)
  line L62 (344.7305, 47.3004) -> (344.7305, 48.3504)
  line L63 (347.664, 48.3504) -> (347.664, 47.3004)
  line L64 (346.8371, 50.6547) -> (346.8371, 48.3504)
  line L65 (346.8371, 47.3004) -> (346.8371, 41.5185)
  line L66 (345.6371, 41.5185) -> (345.6371, 47.3004)
  line L67 (345.6371, 48.3504) -> (345.6371, 50.0608)
  line L68 (347.664, 47.3004) -> (346.8371, 47.3004)
  line L69 (346.5163, 47.4305) -> (346.4947, 47.4305)
  line L70 (344.7305, 48.3504) -> (345.6371, 48.3504)
  line L71 (346.8371, 48.3504) -> (347.664, 48.3504)
  arc A56 (346.8371, 50.6547) -> (344.7026, 50.781) centre (345.6499, 48.6902) ccw
  arc A57 (345.6371, 50.0608) -> (345.0807, 50.1289) centre (345.2418, 49.1368) ccw
  line L72 (345.0807, 50.1289) -> (344.7026, 50.781)
  arc A58 (340.7984, 43.9722) -> (343.6639, 46.4824) centre (340.6109, 47.0769) ccw
  arc A59 (343.6639, 46.4824) -> (340.2476, 50.8652) centre (340.0477, 47.1866) ccw
  arc A60 (340.2476, 50.8652) -> (337.6108, 49.9494) centre (340.0478, 47.1867) ccw
  arc A61 (338.2198, 47.0328) -> (340.7984, 43.9722) centre (340.648, 46.4621) ccw
  arc A62 (340.1979, 49.9497) -> (338.1619, 49.2116) centre (340.0478, 47.1867) ccw
  line L73 (339.4951, 48.0431) -> (342.6791, 48.0431)
  arc A63 (339.4951, 48.0431) -> (338.2198, 47.0328) centre (339.4951, 46.7331) ccw
  arc A64 (342.6791, 48.0431) -> (340.1979, 49.9497) centre (340.0477, 47.1866) ccw
  line L74 (338.1619, 49.2116) -> (337.6108, 49.9494)
  line L75 (336.8119, 50.8649) -> (336.8119, 45.4255)
  line L76 (335.4119, 45.4255) -> (335.4119, 46.0983)
  arc A65 (333.8873, 46.9353) -> (335.4119, 47.4983) centre (334.2311, 48.3499) ccw
  arc A66 (332.6428, 45.7361) -> (335.4119, 46.0983) centre (333.707, 48.3662) ccw
  line L77 (335.4119, 47.4983) -> (335.4119, 50.8649)
  arc A67 (332.8179, 48.2957) -> (333.8873, 46.9353) centre (334.2179, 48.2957) ccw
  arc A68 (331.7679, 47.0339) -> (332.6428, 45.7361) centre (333.1679, 47.0339) ccw
  line L78 (332.8179, 50.8649) -> (332.8179, 48.2957)
  line L79 (331.7679, 47.0339) -> (331.7679, 50.8649)
  line L80 (336.8119, 45.4255) -> (335.4119, 45.4255)
  circle A69 centre (330.6786, 49.5962) radius 0.7
  line L81 (324.4426, 50.8649) -> (324.4426, 41.0649)
  line L82 (324.4426, 41.0649) -> (325.8426, 41.0649)
  line L83 (325.8426, 41.0649) -> (325.8426, 44.646)
  line L84 (325.5578, 50.8608) -> (324.4426, 50.8649)
  arc A70 (325.8426, 44.646) -> (325.5578, 50.8608) centre (325.8426, 47.7599) ccw
  arc A71 (320.1393, 43.9717) -> (323.0044, 46.479) centre (319.9519, 47.0764) ccw
  arc A72 (317.5611, 47.0334) -> (320.1393, 43.9717) centre (319.989, 46.4616) ccw
  arc A73 (318.8362, 48.0431) -> (317.5611, 47.0334) centre (318.8362, 46.7331) ccw
  arc A74 (319.539, 49.9497) -> (317.503, 49.2116) centre (319.3889, 47.1867) ccw
  line L85 (317.503, 49.2116) -> (316.9519, 49.9494)
  arc A75 (319.5888, 50.8652) -> (316.9519, 49.9494) centre (319.3889, 47.1867) ccw
  arc A76 (322.0202, 48.0431) -> (319.539, 49.9497) centre (319.3889, 47.1866) ccw
  arc A77 (323.0044, 46.479) -> (319.5888, 50.8652) centre (319.3889, 47.1866) ccw
  line L86 (318.8362, 48.0431) -> (322.0202, 48.0431)
  line L87 (412.2613, 50.883) -> (409.5613, 50.883)
  line L88 (408.2113, 50.8778) -> (406.4113, 50.8778)
  line L89 (401.5152, 50.8778) -> (398.8152, 50.8778)
  line L90 (368.0691, 50.8649) -> (366.2691, 50.8649)
  line L91 (381.0894, 50.8671) -> (379.9448, 50.8671)
  line L92 (455.7355, 52.5) -> (305.7355, 52.5) projected
  line L93 (375.975, 50.8995) -> (375.1276, 50.8995)
  line L94 (364.8448, 50.8649) -> (363.4448, 50.8649)
  line L95 (360.8509, 50.8649) -> (359.8009, 50.8649)
  line L96 (350.4704, 50.8746) -> (349.0704, 50.8746)
  line L97 (336.8119, 50.8649) -> (335.4119, 50.8649)
  line L98 (332.8179, 50.8649) -> (331.7679, 50.8649)
  line L99 (305.7355, -11) -> (305.7355, 52.5) projected
  line L100 (391.7211, 50.8746) -> (390.6711, 50.8746)
  line L101 (351.0966, 46.1356) -> (351.0966, 50.8032)
  line L102 (394.315, 46.0983) -> (394.315, 41.0746)
  line L103 (395.715, 41.0746) -> (395.715, 50.8746)
  line L104 (395.715, 50.8746) -> (394.315, 50.8746)
  line L105 (394.315, 50.8746) -> (394.315, 47.4983)
  line L106 (379.9448, 50.8671) -> (377.9536, 49.3808)
  line L107 (377.9536, 49.3808) -> (375.975, 50.8995)
  line L108 (380.0718, 49.3006) -> (378.0974, 47.8269)
  line L109 (378.0974, 47.8269) -> (376.1133, 49.3498)
  point P0 (0, 0)
  point P1 (390.6711, 46.295)
  point P2 (391.7211, 48.0001)
  point P3 (369.4934, 48.0431)
  point P4 (369.9696, 47.0764)
  point P5 (359.8009, 46.295)
  point P6 (360.8509, 48.0001)
  point P7 (338.7187, 48.0431)
  point P8 (332.8179, 48.0001)
  point P9 (331.7679, 46.295)
  point P10 (318.5361, 47.0764)
  dimension "d214" = 9
  dimension "d215" = 2.7
  dimension "d216" = 3
  dimension "d218" = 12.6
  dimension "d219" = 1.8
  dimension "d221" = 9
  dimension "d222" = 2.7
  dimension "d223" = 3
  dimension "d224" = 1.35
  dimension "d225" = 1.4
  dimension "d226" = 1.246
  dimension "d227" = 12.0421
  dimension "d229" = 1.4
  dimension "d230" = 1.05
  dimension "d231" = 1.4
  dimension "d232" = 1.4
  dimension "d234" = 1.05
  dimension "d235" = 1.2
  dimension "d236" = 2.8
  dimension "d237" = 1.05
  dimension "d238" = 1
  dimension "d242" = 1
  dimension "d244" = 1.31
  dimension "d247" = 7
  dimension "d248" = 1.8
  dimension "d249" = 1.8
  dimension "d250" = 1.05
  dimension "d251" = 1.4
  dimension "d252" = 1.4
  dimension "d253" = 0.98
  dimension "d257" = 5.6
  dimension "d258" = 1.4
  dimension "d259" = 5.6
  dimension "d261" = 0.84
  dimension "d262" = 1.2
  dimension "d265" = 1.05
  dimension "d266" = 1.05
  dimension "d268" = 1.31
  dimension "d270" = 1.05
  dimension "d271" = 1.4
  dimension "d272" = 1.4
  dimension "d273" = 1.4
  dimension "d274" = 0.776
  dimension "d275" = 0
  dimension "d276" = 0
  dimension "d279" = 9.8
  dimension "d280" = 1.4
  dimension "d281" = 9.8
  dimension "d283" = 1.31
  dimension "d287" = 1.4
  constraints: 216 end point, 154 point on circle, 78 centre point, 27 tangent, 20 perpendicular, 17 vertical, 14 horizontal, 11 point on line, 10 parallel, 3 equal radius, 1 collinear, 3 other
  measures "d214" distance of L0.start L0.end
  measures "d215" distance of L0.end L1.end
  measures "d216" diameter of A0
  measures "d218" distance of L3.start L3.end
  measures "d219" distance of L3.end L4.end
  measures "d221" distance of L11.start L11.end
  measures "d222" distance of L11.end L13.start
  measures "d223" diameter of A1
  measures "d224" distance between parallel lines of L3 L2
  measures "d225" diameter of A2
  measures "d226" distance edge to line of A2 L13
  measures "d229" distance of L16.start L16.end
  measures "d230" distance between parallel lines of L17 L18
  measures "d231" distance of L102.start L105.end
  measures "d232" radius of A5
  measures "d234" radius of A12
  measures "d235" radial gap between concentric circles of A7 A13
  measures "d236" distance of L22.end L23.end
  measures "d237" distance of L21.end L22.end
  measures "d238" distance between parallel lines of L25 L26
  measures "d242" distance between parallel lines of L28 L29
  measures "d244" radius of A23
  measures "d247" distance of L35.start L35.end
  measures "d248" distance of L35.end L34.start
  measures "d249" diameter of A25
  measures "d250" distance between parallel lines of L38 L39
  measures "d251" distance of L40.end L41.start
  measures "d252" radius of A28
  measures "d253" radial gap between concentric circles of A30 A35
  measures "d257" distance of L54.start L54.end
  measures "d258" distance of L54.end L55.end
  measures "d259" distance of L55.end L58.end
  measures "d262" distance of L60.start L60.end
  measures "d265" distance of L61.end L62.end
  measures "d266" distance of L63.start L63.end
  measures "d268" radius of A63
  measures "d270" distance between parallel lines of L79 L78
  measures "d271" distance of L76.end L77.start
  measures "d272" radius of A67
  measures "d273" diameter of A69
  measures "d274" distance between parallel lines of L65 L56
  measures "d275" distance between parallel lines of L64 L65
  measures "d276" distance between parallel lines of L66 L67
  measures "d279" distance of L81.start L81.end
  measures "d280" distance of L81.end L82.end
  measures "d281" distance of L82.end L84.start
  measures "d283" radius of A73
  measures "d287" distance of L103.end L104.end
extrude "Extrusion12" add sketch "Sketch13" along normal blind 3 contours L0 L1 L2 L87 | A0 | L3 L4 L14 L5 L6 L7 L10 L9 L8 L15 L88 | L11 L12 L13 L89 | A1 | A2 | L16 L102 A3 A6 L17 L100 L18 A5 A4 L105 L104 L103 | L20 A13 A14 A15 A16 A17 L19 A8 A10 A12 A9 A11 A7 | L21 L22 L23 L24 | L30 L26 L108 L109 L29 L31 L28 L93 L107 L106 L91 L25 | A21 A23 L32 A24 A22 L33 A20 A19 A18 | L34 L90 L35 L36 | A25 | L37 L42 L40 A26 A29 L38 L95 L39 A28 A27 L41 L94 | A31 A32 L43 A33 A34 L48 A52 A51 L45 A39 A30 | A36 A37 L44 A38 A35 | A42 L46 A41 A46 A40 | A47 L47 A48 A49 L49 L53 L50 A53 A50 L101 L52 L51 A45 A44 A43 | L54 L55 L57 L59 A54 L56 A55 L58 L96 | L60 L66 L61 L62 L70 L67 A57 L72 A56 L64 L71 L63 L68 L65 | A61 A63 L73 A64 A62 L74 A60 A59 A58 | L75 L80 L76 A66 A68 L79 L98 L78 A67 A65 L77 L97 | A69 | L84 A70 L83 L82 L81 | A72 A73 L86 A76 A74 L85 A75 A77 A71
sketch "Sketch15" plane through (7, 0, 0) normal (1, 0, 0) x (0, 0, -1)
  line L0 (455.7355, -36.5) -> (455.7355, 36.5)
  line L1 (453.2355, -20) -> (413.6355, -20)
  line L2 (453.2355, 20) -> (413.6355, 20)
  circle A0 centre (413.6355, -20) radius 0.75
  circle A1 centre (413.6355, 20) radius 0.75
  circle A2 centre (453.2355, 20) radius 0.75
  circle A3 centre (453.2355, -20) radius 0.75
  circle A4 centre (453.2355, 0) radius 0.75
  circle A5 centre (413.6355, 0) radius 0.75
  point P0 (0, 0)
  dimension "d296" = 1.5
  dimension "d297" = 1.5
  dimension "d298" = 1.5
  dimension "d299" = 1.5
  dimension "d300" = 1.5
  dimension "d301" = 1.5
  constraints: 6 centre point, 6 end point, 4 coincident, 1 vertical
  measures "d296" diameter of A0
  measures "d297" diameter of A1
  measures "d298" diameter of A2
  measures "d299" diameter of A3
  measures "d300" diameter of A4
  measures "d301" diameter of A5
extrude "Extrusion13" cut sketch "Sketch15" against normal blind 10
body "Solid1"
